sunburst (Autodesk Fusion 360 design; units mm, degrees)
Autodesk Fusion 360 part; units mm, degrees
extrude "Extrude6" [suppressed]
ref_plane "WorkPlane1" through (-0.7494, -0.6, 4.8151) normal (0, -1, 0) x (0, 0, -1)
sketch "Sketch3" plane through (0, -0.6, 0) normal (0, -1, 0) x (-1, 0, 0)
  circle A0 centre (0, 0) radius 28
  dimension "d32" = 56
  constraint coincident A0.centre origin
  measures "d32" diameter of A0
extrude "Extrude7" [suppressed]
sketch "sketch 197" plane through (0, 0, 0) normal (0, 1, 0) x (1, 0, 0)
  circle A0 centre (0, 0) radius 5
  circle A1 centre (0, 0) radius 6
  circle A2 centre (0, 0) radius 16
  circle A3 centre (0, 0) radius 17
  circle A4 centre (0, 0) radius 26.5
  circle A5 centre (0, 0) radius 27.5
  circle A6 centre (0, 0) radius 33
  line L0 (-3.9046, 4.5557) -> (-9.6929, 12.7298)
  line L1 (-5.6565, 2.001) -> (-15.1209, 5.2305)
  line L2 (-16.1216, 5.3938) -> (-25.1127, 8.4617)
  line L3 (-24.375, 10.3976) -> (-15.6425, 6.6566)
  line L4 (-15.4468, 7.0991) -> (-24.0905, 11.0407)
  line L5 (-15.0805, 7.8473) -> (-23.43, 12.3808)
  line L6 (-14.8296, 8.3116) -> (-23.1046, 12.9779)
  line L7 (-22.3505, 14.2374) -> (-14.3911, 9.0497)
  line L8 (-14.0817, 9.524) -> (-21.9358, 14.8684)
  line L9 (-20.5642, 16.7142) -> (-13.2548, 10.6447)
  line L10 (-26.5492, 7.1686) -> (-31.8756, 8.5408)
  line L11 (-31.236, 10.6447) -> (-26.0698, 8.7529)
  line L12 (-25.8745, 9.3144) -> (-31.0392, 11.2056)
  line L13 (-30.2541, 13.1791) -> (-25.2442, 10.9077)
  line L14 (-5.8159, 1.4749) -> (-15.3347, 4.5657)
  line L15 (-5.9819, -0.4663) -> (-15.8908, -1.8658)
  line L16 (-5.8856, -1.166) -> (-15.7623, -2.7475)
  line L17 (-3.2548, -5.0405) -> (-8.4775, -13.5695)
  line L18 (-7.87, -13.9307) -> (-2.6391, -5.3884)
  line L19 (0.3065, -5.9922) -> (1.4776, -15.9316)
  line L20 (2.4796, -15.8067) -> (1.09, -5.9002)
  line L21 (2.2431, -5.5649) -> (6.8423, -14.4632)
  line L22 (7.5569, -14.103) -> (2.964, -5.2168)
  line L23 (5.7898, 1.5741) -> (15.2163, 4.9462)
  line L24 (14.9323, 5.7469) -> (5.5751, 2.2176)
  line L25 (12.3522, 10.1697) -> (4.8981, 3.4653)
  line L26 (4.2215, 4.2636) -> (11.6613, 10.9551)
  line L27 (1.1172, 5.8951) -> (3.7964, 15.5431)
  line L28 (4.6866, 15.2982) -> (2.0085, 5.6538)
  line L29 (-3.1659, 5.0968) -> (-8.9039, 13.2936)
  line L30 (-16.5713, 3.7935) -> (-25.8898, 5.6538)
  line L31 (-16.3375, 4.6995) -> (-25.3936, 7.5771)
  line L32 (-26.399, 2.3114) -> (-16.9218, 1.6288)
  line L33 (-26.045, 4.8897) -> (-16.7279, 3.0296)
  line L34 (-26.4638, 1.3844) -> (-16.9855, 0.7017)
  line L35 (-26.2905, -3.3257) -> (-16.8977, -1.8621)
  line L36 (-26.191, -4.0353) -> (-16.7685, -2.7959)
  line L37 (-25.7871, -6.1054) -> (-16.5831, -3.742)
  line L38 (-7.4849, -25.421) -> (-4.6905, -16.3401)
  line L39 (-5.7669, -25.8649) -> (-3.8484, -16.5587)
  line L40 (0, -26.5) -> (0, -17)
  line L41 (-2.951, -16.7419) -> (-4.8696, -26.0487)
  line L42 (0.8661, -26.4858) -> (0.6304, -16.9883)
  line L43 (1.8311, -16.9011) -> (2.9765, -26.3323)
  line L44 (6.0603, -25.7977) -> (4.0068, -16.5211)
  line L45 (5.3634, -16.1318) -> (8.5144, -25.0949)
  line L46 (9.4324, -24.7645) -> (6.1019, -15.8672)
  line L47 (11.7605, -23.7474) -> (7.3572, -15.3255)
  line L48 (12.6046, -23.3104) -> (8.2022, -14.8904)
  line L49 (9.0465, -14.3931) -> (14.3256, -22.2941)
  line L50 (9.7988, -13.8918) -> (15.1912, -21.7135)
  line L51 (10.2957, -13.5277) -> (16.3371, -20.865)
  line L52 (11.0727, -12.8994) -> (17.1122, -20.2342)
  line L53 (11.8744, -12.1655) -> (18.6003, -18.8753)
  line L54 (13.7033, -10.0608) -> (21.1773, -15.9303)
  line L55 (15.9319, -5.9308) -> (24.934, -8.9747)
  line L56 (16.2213, -5.0862) -> (25.2771, -7.9572)
  line L57 (16.8901, -1.9298) -> (26.3655, -2.6665)
  line L58 (16.9669, -1.0605) -> (26.439, -1.797)
  line L59 (16.9902, 0.5773) -> (26.4772, 1.0989)
  line L60 (26.4135, 2.1398) -> (16.9358, 1.4761)
  line L61 (16.6138, 3.6031) -> (25.8333, 5.9067)
  line L62 (25.6212, 6.7677) -> (16.4033, 4.4645)
  line L63 (16.1363, 5.3498) -> (25.0535, 8.6356)
  line L64 (24.6784, 9.6554) -> (15.8245, 6.2117)
  line L65 (15.4197, 7.1577) -> (24.0445, 11.1406)
  line L66 (23.7354, 11.7848) -> (15.2099, 7.5934)
  line L67 (14.795, 8.373) -> (23.0554, 13.0652)
  line L68 (22.5, 14) -> (14.328, 9.1492)
  line L69 (21.2388, 15.8482) -> (13.553, 10.2623)
  line L70 (12.1982, 11.8408) -> (19.1494, 18.3181)
  line L71 (18.0736, 19.3803) -> (11.621, 12.4078)
  line L72 (11.1445, 12.8374) -> (17.6399, 19.7758)
  line L73 (16.0889, 21.057) -> (10.3305, 13.5011)
  line L74 (9.878, 13.8356) -> (15.6381, 21.3939)
  line L75 (14.6155, 22.1051) -> (9.3319, 14.2097)
  line L76 (7.3498, 15.3291) -> (11.7201, 23.7674)
  line L77 (9.9713, 24.5525) -> (6.3491, 15.7699)
  line L78 (9.2924, 24.8174) -> (5.8178, 15.9735)
  line L79 (7.4164, 25.4411) -> (4.7967, 16.3092)
  line L80 (6.3491, 25.7282) -> (3.8859, 16.5499)
  line L81 (3.8859, 26.2135) -> (2.6171, 16.7973)
  line L82 (3.1138, 26.3164) -> (1.8449, 16.8996)
  line L83 (1.2408, 26.4709) -> (0.92, 16.9751)
  line L84 (0.6334, 26.4924) -> (0.3127, 16.9971)
  line L85 (-1.1755, 26.4739) -> (-0.8096, 16.9807)
  line L86 (-1.8148, 26.4378) -> (-1.4486, 16.9382)
  line L87 (-4.2572, 26.1558) -> (-2.5895, 16.8016)
  line L88 (-4.9119, 26.0408) -> (-3.4233, 16.6518)
  line L89 (-6.7746, 25.6194) -> (-4.3029, 16.4464)
  line L90 (-7.4272, 25.4379) -> (-4.6925, 16.3395)
  line L91 (-8.6485, 25.049) -> (-5.5387, 16.0724)
  line L92 (-9.2604, 24.8293) -> (-5.9347, 15.9305)
  line L93 (-10.5439, 24.3121) -> (-6.7389, 15.6073)
  line L94 (-11.0798, 24.0726) -> (-7.2737, 15.3653)
  line L95 (-12.5073, 23.3627) -> (-8, 15)
  line L96 (-13.1462, 23.0093) -> (-8.446, 14.7535)
  line L97 (-15.2182, 21.6946) -> (-9.5864, 14.0392)
  line L98 (-15.9612, 21.1539) -> (-10.331, 13.5007)
  line L99 (-17.5978, 19.8133) -> (-11.2411, 12.7529)
  line L100 (-23.1855, 23.4826) -> (-19.2651, 19.6242)
  line L101 (-22.1696, 24.444) -> (-18.4895, 20.3566)
  line L102 (-21.5449, 24.9963) -> (-17.8638, 20.9078)
  line L103 (-20.5857, 25.792) -> (-17.0793, 21.5534)
  line L104 (-17.9748, 27.675) -> (-14.8657, 23.1357)
  line L105 (-16.2704, 28.7101) -> (-13.6536, 23.8711)
  line L106 (-15.7952, 28.9743) -> (-13.0339, 24.215)
  line L107 (-14.0759, 29.8474) -> (-11.7698, 24.854)
  line L108 (-10.616, 31.2458) -> (-8.8282, 26.0444)
  line L109 (-9.5266, 31.595) -> (-7.9766, 26.3178)
  line L110 (-8.6438, 31.8478) -> (-7.1988, 26.5411)
  line L111 (-7.5092, 32.1343) -> (-6.3363, 26.7601)
  line L112 (-0.704, 32.9925) -> (-0.5292, 27.4949)
  line L113 (0.5327, 32.9957) -> (0.4096, 27.4969)
  line L114 (1.4606, 32.9677) -> (1.1772, 27.4748)
  line L115 (2.6616, 32.8925) -> (2.1566, 27.4153)
  line L116 (13.4068, 30.1539) -> (11.1032, 25.1589)
  line L117 (12.255, 24.6184) -> (14.8392, 29.4754)
  line L118 (25.4963, 20.9509) -> (21.1963, 17.5204)
  line L119 (22.3915, 15.9647) -> (26.814, 19.2357)
  line L120 (30.5346, 12.5156) -> (25.4747, 10.3581)
  line L121 (25.8193, 9.4666) -> (30.9951, 11.3272)
  line L122 (31.7345, 9.0509) -> (26.4504, 7.5251)
  line L123 (26.7308, 6.4588) -> (32.0505, 7.8593)
  line L124 (32.5136, 5.6451) -> (27.1002, 4.6722)
  line L125 (27.2454, 3.7332) -> (32.6896, 4.5156)
  line L126 (32.7629, 3.9486) -> (27.2995, 3.3149)
  line L127 (27.3861, 2.5002) -> (32.8643, 2.9897)
  line L128 (32.9337, 2.0913) -> (27.4395, 1.8225)
  line L129 (27.4849, 0.9123) -> (32.9874, 0.9123)
  line L130 (32.9822, -1.085) -> (27.4849, -0.9117)
  line L131 (27.4395, -1.8225) -> (32.9306, -2.1396)
  line L132 (32.7757, -3.8411) -> (27.3199, -3.1425)
  line L133 (27.1875, -4.1342) -> (32.6082, -5.07)
  line L134 (5.5375, -32.5321) -> (4.6, -27.1125)
  line L135 (3.5952, -27.264) -> (4.2286, -32.728)
  line L136 (3.0895, -27.3259) -> (3.6634, -32.796)
  line L137 (2.669, -32.8919) -> (2.3996, -27.3951)
  line L138 (2.2276, -32.9247) -> (1.8643, -27.4367)
  line L139 (1.2645, -32.9758) -> (1.0932, -27.4783)
  line L140 (0.7707, -32.991) -> (0.5994, -27.4935)
  line L141 (-0.9829, -32.9854) -> (-0.8607, -27.4865)
  line L142 (-1.7716, -32.9524) -> (-1.5108, -27.4585)
  line L143 (-4.0581, -32.7495) -> (-3.3505, -27.2951)
  line L144 (-30.3823, -12.8808) -> (-25.4093, -10.5174)
  line L145 (-26.1354, -8.5552) -> (-31.4006, -10.1491)
  line L146 (-26.3937, -7.7215) -> (-31.6471, -9.3522)
  line L147 (-26.6921, -6.6169) -> (-32.0193, -7.9853)
  line L148 (-26.8427, -5.9766) -> (-32.2121, -7.1681)
  line L149 (-27.1016, -4.6639) -> (-32.5055, -5.6915)
  constraint coincident A0.centre A1.centre
  constraint concentric A0 A1
  constraint concentric A1 A2
  constraint concentric A1 A3
  constraint concentric A3 A5
  constraint concentric A4 A6
  constraint coincident A1 L0.start
  constraint coincident A2 L0.end
  constraint coincident A1 L1.start
  constraint coincident A2 L1.end
  constraint coincident A3 L2.start
  constraint coincident A4 L2.end
  constraint parallel L1 L2
  constraint coincident A4 L3.start
  constraint coincident A3 L3.end
  constraint coincident A3 L4.start
  constraint coincident A4 L4.end
  constraint coincident A3 L5.start
  constraint coincident A4 L5.end
  constraint coincident A3 L6.start
  constraint coincident A4 L6.end
  constraint coincident A4 L7.start
  constraint coincident A3 L7.end
  constraint coincident A3 L8.start
  constraint coincident A4 L8.end
  constraint coincident A4 L9.start
  constraint coincident A3 L9.end
  constraint coincident A5 L10.start
  constraint coincident A6 L10.end
  constraint coincident A6 L11.start
  constraint coincident A5 L11.end
  constraint coincident A5 L12.start
  constraint coincident A6 L12.end
  constraint parallel L11 L12
  constraint coincident A6 L13.start
  constraint coincident A5 L13.end
  constraint coincident A1 L14.start
  constraint coincident A2 L14.end
  constraint coincident A1 L15.start
  constraint coincident A2 L15.end
  constraint coincident A1 L16.start
  constraint coincident A2 L16.end
  constraint coincident A1 L17.start
  constraint coincident A2 L17.end
  constraint coincident A2 L18.start
  constraint coincident A1 L18.end
  constraint parallel L17 L18
  constraint coincident A1 L19.start
  constraint coincident A2 L19.end
  constraint coincident A2 L20.start
  constraint coincident A1 L20.end
  constraint coincident A1 L21.start
  constraint coincident A2 L21.end
  constraint coincident A2 L22.start
  constraint coincident A1 L22.end
  constraint parallel L21 L22
  constraint coincident A1 L23.start
  constraint coincident A2 L23.end
  constraint coincident A2 L24.start
  constraint coincident A1 L24.end
  constraint coincident A2 L25.start
  constraint coincident A1 L25.end
  constraint coincident A1 L26.start
  constraint coincident A2 L26.end
  constraint parallel L25 L26
  constraint coincident A1 L27.start
  constraint coincident A2 L27.end
  constraint coincident A2 L28.start
  constraint coincident A1 L28.end
  constraint parallel L27 L28
  constraint coincident A1 L29.start
  constraint coincident A2 L29.end
  constraint coincident A3 L30.start
  constraint coincident A4 L30.end
  constraint coincident A3 L31.start
  constraint coincident A4 L31.end
  constraint coincident A4 L32.start
  constraint coincident A3 L32.end
  constraint coincident A4 L33.start
  constraint coincident A3 L33.end
  constraint parallel L30 L33
  constraint coincident A4 L34.start
  constraint coincident A3 L34.end
  constraint parallel L32 L34
  constraint coincident A4 L35.start
  constraint coincident A3 L35.end
  constraint coincident A4 L36.start
  constraint coincident A3 L36.end
  constraint coincident A4 L37.start
  constraint coincident A3 L37.end
  constraint coincident A4 L38.start
  constraint coincident A3 L38.end
  constraint coincident A4 L39.start
  constraint coincident A3 L39.end
  constraint coincident A4 L40.start
  constraint coincident A3 L40.end
  constraint vertical L40
  constraint coincident A3 L41.start
  constraint coincident A4 L41.end
  constraint parallel L39 L41
  constraint coincident A4 L42.start
  constraint coincident A3 L42.end
  constraint coincident A3 L43.start
  constraint coincident A4 L43.end
  constraint coincident A4 L44.start
  constraint coincident A3 L44.end
  constraint coincident A3 L45.start
  constraint coincident A4 L45.end
  constraint coincident A4 L46.start
  constraint coincident A3 L46.end
  constraint coincident A4 L47.start
  constraint coincident A3 L47.end
  constraint coincident A4 L48.start
  constraint coincident A3 L48.end
  constraint parallel L47 L48
  constraint coincident A3 L49.start
  constraint coincident A4 L49.end
  constraint coincident A3 L50.start
  constraint coincident A4 L50.end
  constraint coincident A3 L51.start
  constraint coincident A4 L51.end
  constraint coincident A3 L52.start
  constraint coincident A4 L52.end
  constraint parallel L51 L52
  constraint coincident A3 L53.start
  constraint coincident A4 L53.end
  constraint coincident A3 L54.start
  constraint coincident A4 L54.end
  constraint coincident A3 L55.start
  constraint coincident A4 L55.end
  constraint coincident A3 L56.start
  constraint coincident A4 L56.end
  constraint coincident A3 L57.start
  constraint coincident A4 L57.end
  constraint coincident A3 L58.start
  constraint coincident A4 L58.end
  constraint parallel L57 L58
  constraint coincident A3 L59.start
  constraint coincident A4 L59.end
  constraint coincident A3 L60.end
  constraint coincident A3 L61.start
  constraint coincident A4 L61.end
  constraint coincident A4 L62.start
  constraint coincident A3 L62.end
  constraint parallel L61 L62
  constraint coincident A3 L63.start
  constraint coincident A4 L63.end
  constraint coincident A4 L64.start
  constraint coincident A3 L64.end
  constraint coincident A3 L65.start
  constraint coincident A4 L65.end
  constraint coincident A4 L66.start
  constraint coincident A3 L66.end
  constraint coincident A3 L67.start
  constraint coincident A4 L67.end
  constraint coincident A4 L68.start
  constraint coincident A3 L68.end
  constraint coincident A4 L69.start
  constraint coincident A3 L69.end
  constraint coincident A3 L70.start
  constraint coincident A4 L70.end
  constraint coincident A4 L71.start
  constraint coincident A3 L71.end
  constraint coincident A3 L72.start
  constraint coincident A4 L72.end
  constraint coincident A4 L73.start
  constraint coincident A3 L73.end
  constraint coincident A3 L74.start
  constraint coincident A4 L74.end
  constraint parallel L73 L74
  constraint coincident A4 L75.start
  constraint coincident A3 L75.end
  constraint coincident A3 L76.start
  constraint coincident A4 L76.end
  constraint coincident A4 L77.start
  constraint coincident A3 L77.end
  constraint coincident A4 L78.start
  constraint coincident A3 L78.end
  constraint coincident A4 L79.start
  constraint coincident A3 L79.end
  constraint coincident A4 L80.start
  constraint coincident A3 L80.end
  constraint coincident A4 L81.start
  constraint coincident A3 L81.end
  constraint coincident A4 L82.start
  constraint coincident A3 L82.end
  constraint parallel L81 L82
  constraint coincident A4 L83.start
  constraint coincident A3 L83.end
  constraint coincident A4 L84.start
  constraint coincident A3 L84.end
  constraint parallel L83 L84
  constraint coincident A4 L85.start
  constraint coincident A3 L85.end
  constraint coincident A4 L86.start
  constraint coincident A3 L86.end
  constraint parallel L85 L86
  constraint coincident A4 L87.start
  constraint coincident A3 L87.end
  constraint coincident A4 L88.start
  constraint coincident A3 L88.end
  constraint coincident A4 L89.start
  constraint coincident A3 L89.end
  constraint coincident A4 L90.start
  constraint coincident A3 L90.end
  constraint coincident A4 L91.start
  constraint coincident A3 L91.end
  constraint coincident A4 L92.start
  constraint coincident A3 L92.end
  constraint coincident A4 L93.start
  constraint coincident A3 L93.end
  constraint coincident A4 L94.start
  constraint coincident A3 L94.end
  constraint parallel L93 L94
  constraint coincident A4 L95.start
  constraint coincident A3 L95.end
  constraint coincident A4 L96.start
  constraint coincident A3 L96.end
  constraint coincident A4 L97.start
  constraint coincident A3 L97.end
  constraint coincident A4 L98.start
  constraint coincident A3 L98.end
  constraint parallel L97 L98
  constraint coincident A4 L99.start
  constraint coincident A3 L99.end
  constraint coincident A6 L100.start
  constraint coincident A5 L100.end
  constraint coincident A6 L101.start
  constraint coincident A5 L101.end
  constraint parallel L99 L101
  constraint coincident A6 L102.start
  constraint coincident A5 L102.end
  constraint parallel L101 L102
  constraint coincident A6 L103.start
  constraint coincident A5 L103.end
  constraint coincident A6 L104.start
  constraint coincident A5 L104.end
  constraint coincident A6 L105.start
  constraint coincident A5 L105.end
  constraint coincident A6 L106.start
  constraint coincident A5 L106.end
  constraint coincident A6 L107.start
  constraint coincident A5 L107.end
  constraint coincident A6 L108.start
  constraint coincident A5 L108.end
  constraint coincident A6 L109.start
  constraint coincident A5 L109.end
  constraint coincident A6 L110.start
  constraint coincident A5 L110.end
  constraint coincident A6 L111.start
  constraint coincident A5 L111.end
  constraint coincident A6 L112.start
  constraint coincident A5 L112.end
  constraint coincident A6 L113.start
  constraint coincident A5 L113.end
  constraint coincident A6 L114.start
  constraint coincident A5 L114.end
  constraint coincident A6 L115.start
  constraint coincident A5 L115.end
  constraint coincident A6 L116.start
  constraint coincident A5 L116.end
  constraint coincident A5 L117.start
  constraint coincident A6 L117.end
  constraint coincident A6 L118.start
  constraint coincident A5 L118.end
  constraint coincident A5 L119.start
  constraint coincident A6 L119.end
  constraint coincident A6 L120.start
  constraint coincident A5 L120.end
  constraint coincident A5 L121.start
  constraint coincident A6 L121.end
  constraint coincident A6 L122.start
  constraint coincident A5 L122.end
  constraint coincident A5 L123.start
  constraint coincident A6 L123.end
  constraint coincident A6 L124.start
  constraint coincident A5 L124.end
  constraint coincident A5 L125.start
  constraint coincident A6 L125.end
  constraint coincident A6 L126.start
  constraint coincident A5 L126.end
  constraint coincident A5 L127.start
  constraint coincident A6 L127.end
  constraint coincident A6 L128.start
  constraint coincident A5 L128.end
  constraint coincident A6 L129.end
  constraint horizontal L129
  constraint coincident A6 L130.start
  constraint coincident A5 L130.end
  constraint coincident A5 L131.start
  constraint coincident A6 L131.end
  constraint coincident A6 L132.start
  constraint coincident A5 L132.end
  constraint coincident A5 L133.start
  constraint coincident A6 L133.end
  constraint coincident A6 L134.start
  constraint coincident A5 L134.end
  constraint coincident A5 L135.start
  constraint coincident A6 L135.end
  constraint coincident A5 L136.start
  constraint coincident A6 L136.end
  constraint coincident A6 L137.start
  constraint coincident A5 L137.end
  constraint coincident A6 L138.start
  constraint coincident A5 L138.end
  constraint coincident A6 L139.start
  constraint coincident A5 L139.end
  constraint coincident A6 L140.start
  constraint coincident A5 L140.end
  constraint parallel L139 L140
  constraint coincident A5 L141.end
  constraint coincident A6 L142.start
  constraint coincident A5 L142.end
  constraint coincident A6 L143.start
  constraint coincident A5 L143.end
  constraint coincident A6 L144.start
  constraint coincident A5 L144.end
  constraint coincident A5 L145.start
  constraint coincident A6 L145.end
  constraint coincident A5 L146.start
  constraint coincident A6 L146.end
  constraint coincident A5 L147.start
  constraint coincident A6 L147.end
  constraint coincident A5 L148.start
  constraint coincident A6 L148.end
  constraint coincident A5 L149.start
  constraint coincident A6 L149.end
  constraint coincident A6 L141.start
  constraint coincident A5 L129.start
  constraint coincident A4 L60.start
  measures "d1" diameter of A0
  measures "d2" diameter of A1
  measures "d3" diameter of A2
  measures "d4" diameter of A3
  measures "d5" diameter of A4
  measures "d6" diameter of A5
  measures "d7" diameter of A6
extrude "Extrude8" add sketch "sketch 197" against normal blind 1.8 contours A0 | A1 | A1 A2 L22 L23 | A1 A2 L23 L24 | A1 A2 L21 L22 | A1 A2 L24 L25 | A1 A2 L20 L21 | A1 A2 L25 L26 | A1 A2 L19 L20 | A1 A2 L26 L28 | A1 A2 L18 L19 | A1 A2 L27 L28 | A1 A2 L17 L18 | A1 A2 L27 L29 | A1 A2 L16 L17 | A1 A2 L0 L29 | A1 A2 L15 L16 | A1 A2 L0 L1 | A1 A2 L14 L15 | A1 A2 L1 L14 | A3 | A3 A4 L58 L59 | A3 A4 L59 L60 | A3 A4 L57 L58 | A3 A4 L60 L61 | A3 A4 L56 L57 | A3 A4 L61 L62 | A3 A4 L55 L56 | A3 A4 L62 L63 | A3 A4 L54 L55 | A3 A4 L63 L64 | A3 A4 L53 L54 | A3 A4 L64 L65 | A3 A4 L52 L53 | A3 A4 L65 L66 | A3 A4 L51 L52 | A3 A4 L66 L67 | A3 A4 L50 L51 | A3 A4 L67 L68 | A3 A4 L49 L50 | A3 A4 L68 L69 | A3 A4 L48 L49 | A3 A4 L69 L70 | A3 A4 L47 L48 | A3 A4 L70 L71 | A3 A4 L46 L47 | A3 A4 L71 L72 | A3 A4 L45 L46 | A3 A4 L72 L73 | A3 A4 L44 L45 | A3 A4 L73 L74 | A3 A4 L43 L44 | A3 A4 L74 L75 | A3 A4 L42 L43 | A3 A4 L75 L76 | A3 A4 L40 L42 | A3 A4 L76 L77 | A3 A4 L40 L41 | A3 A4 L77 L78 | A3 A4 L39 L41 | A3 A4 L78 L79 | A3 A4 L38 L39 | A3 A4 L79 L80 | A3 A4 L37 L38 | A3 A4 L80 L81 | A3 A4 L36 L37 | A3 A4 L81 L82 | A3 A4 L35 L36 | A3 A4 L82 L83 | A3 A4 L34 L35 | A3 A4 L83 L84 | A3 A4 L32 L34 | A3 A4 L84 L85 | A3 A4 L32 L33 | A3 A4 L85 L86 | A3 A4 L30 L33 | A3 A4 L86 L87 | A3 A4 L30 L31 | A3 A4 L87 L88 | A3 A4 L2 L31 | A3 A4 L88 L89 | A3 A4 L2 L3 | A3 A4 L89 L90 | A3 A4 L3 L4 | A3 A4 L90 L91 | A3 A4 L4 L5 | A3 A4 L91 L92 | A3 A4 L5 L6 | A3 A4 L92 L93 | A3 A4 L6 L7 | A3 A4 L93 L94 | A3 A4 L7 L8 | A3 A4 L94 L95 | A3 A4 L8 L9 | A3 A4 L95 L96 | A3 A4 L9 L99 | A3 A4 L96 L97 | A3 A4 L98 L99 | A3 A4 L97 L98 | A5 | A5 A6 L129 L130 | A5 A6 L128 L129 | A5 A6 L130 L131 | A5 A6 L127 L128 | A5 A6 L131 L132 | A5 A6 L126 L127 | A5 A6 L132 L133 | A5 A6 L125 L126 | A5 A6 L133 L134 | A5 A6 L124 L125 | A5 A6 L134 L135 | A5 A6 L123 L124 | A5 A6 L135 L136 | A5 A6 L122 L123 | A5 A6 L136 L137 | A5 A6 L121 L122 | A5 A6 L137 L138 | A5 A6 L120 L121 | A5 A6 L138 L139 | A5 A6 L119 L120 | A5 A6 L139 L140 | A5 A6 L118 L119 | A5 A6 L140 L141 | A5 A6 L117 L118 | A5 A6 L141 L142 | A5 A6 L116 L117 | A5 A6 L142 L143 | A5 A6 L115 L116 | A5 A6 L143 L144 | A5 A6 L114 L115 | A5 A6 L144 L145 | A5 A6 L113 L114 | A5 A6 L145 L146 | A5 A6 L112 L113 | A5 A6 L146 L147 | A5 A6 L111 L112 | A5 A6 L147 L148 | A5 A6 L110 L111 | A5 A6 L148 L149 | A5 A6 L109 L110 | A5 A6 L10 L149 | A5 A6 L108 L109 | A5 A6 L10 L11 | A5 A6 L107 L108 | A5 A6 L11 L12 | A5 A6 L106 L107 | A5 A6 L12 L13 | A5 A6 L105 L106 | A5 A6 L13 L100 | A5 A6 L104 L105 | A5 A6 L100 L101 | A5 A6 L103 L104 | A5 A6 L101 L102 | A5 A6 L102 L103 makes body 1
extrude "Extrude1" add sketch "sketch 197" along normal blind 1 separate body contours A1 A2 L18 L19 | A1 A2 L27 L29 | A1 A2 L16 L17 | A1 A2 L0 L1 | A1 A2 L14 L15 makes body 2 at (-12.3205, 0, -2.8314) makes body 3 at (-12.2909, 0, 2.9444) makes body 4 at (-8.3492, 0, -9.4871) makes body 5 at (-5.545, 0, 11.3667) makes body 6 at (-1.347, 0, -12.5692) in component "Ring 0 - pro"
extrude "Extrude1'" add sketch "sketch 197" along normal blind 1 separate body contours A1 A2 L22 L23 | A1 A2 L24 L25 | A1 A2 L20 L21 | A1 A2 L26 L28 makes body 7 at (12.451, 0, 2.1821) makes body 8 at (10.9191, 0, -6.3897) makes body 9 at (4.8395, 0, 11.6925) makes body 10 at (5.9656, 0, -11.1484) in component "Ring 0 - con"
extrude "Extrude1''" add sketch "sketch 197" along normal blind 0.8 separate body contours A3 A4 L58 L59 | A3 A4 L60 L61 | A3 A4 L66 L67 | A3 A4 L68 L69 | A3 A4 L46 L47 | A3 A4 L42 L43 | A3 A4 L76 L77 | A3 A4 L40 L41 | A3 A4 L78 L79 | A3 A4 L36 L37 | A3 A4 L34 L35 | A3 A4 L32 L33 | A3 A4 L88 L89 | A3 A4 L2 L3 | A3 A4 L90 L91 | A3 A4 L4 L5 | A3 A4 L92 L93 | A3 A4 L6 L7 | A3 A4 L94 L95 | A3 A4 L8 L9 | A3 A4 L96 L97 makes body 11 at (-23.21, 0, -2.3716) makes body 12 at (-18.286, 0, -14.4904) makes body 13 at (-6.7465, 0, -22.3361) makes body 14 at (19.6417, 0, -12.5923) makes body 15 at (10.0377, 0, 21.0614) makes body 16 at (2.3607, 0, 23.2119) makes body 17 at (20.8206, 0, -10.5313) makes body 18 at (-5.137, 0, -22.7595) makes body 19 at (-13.1153, 0, -19.296) makes body 20 at (-21.9898, 0, -7.798) makes body 21 at (-23.2099, 0, 2.3159) makes body 22 at (-19.7838, 0, -12.3698) makes body 23 at (-9.134, 0, -21.4704) makes body 24 at (10.0711, 0, -21.0465) makes body 25 at (23.3224, 0, -0.6032) makes body 26 at (-3.6924, 0, 23.0299) makes body 27 at (22.8447, 0, -4.7235) makes body 28 at (7.9275, 0, -21.9439) makes body 29 at (-9.9713, 0, -21.0945) makes body 30 at (-20.723, 0, -10.7221) makes body 31 at (-23.0114, 0, 3.8533) in component "Ring 1 - pro"
extrude "Extrude1'''" add sketch "sketch 197" along normal blind 0.8 separate body contours A3 A4 L56 L57 | A3 A4 L62 L63 | A3 A4 L54 L55 | A3 A4 L64 L65 | A3 A4 L52 L53 | A3 A4 L50 L51 | A3 A4 L48 L49 | A3 A4 L70 L71 | A3 A4 L72 L73 | A3 A4 L44 L45 | A3 A4 L74 L75 | A3 A4 L38 L39 | A3 A4 L80 L81 | A3 A4 L82 L83 | A3 A4 L84 L85 | A3 A4 L86 L87 | A3 A4 L30 L31 | A3 A4 L98 L99 makes body 32 at (-1.965, 0, -23.2483) makes body 33 at (13.3196, 0, -19.1575) makes body 34 at (22.1492, 0, -7.3344) makes body 35 at (13.89, 0, 18.7478) makes body 36 at (-5.3194, 0, 22.7178) makes body 37 at (15.2682, 0, 17.6425) makes body 38 at (21.66, 0, -8.6739) makes body 39 at (5.2561, 0, -22.7313) makes body 40 at (-14.2703, 0, -18.4588) makes body 41 at (0.3255, 0, -23.3298) makes body 42 at (15.3061, 0, -17.6097) makes body 43 at (23.1262, 0, 3.0166) makes body 44 at (12.3775, 0, 19.7782) makes body 45 at (5.651, 0, 22.6362) makes body 46 at (19.1799, 0, 13.244) makes body 47 at (16.715, 0, -16.2793) makes body 48 at (2.4832, 0, -23.1996) makes body 49 at (-22.7339, 0, -5.2488) in component "Ring 1 - con"
extrude "Extrude1''''" add sketch "sketch 197" along normal blind 0.4 separate body contours A5 A6 L128 L129 | A5 A6 L130 L131 | A5 A6 L134 L135 | A5 A6 L136 L137 | A5 A6 L118 L119 | A5 A6 L114 L115 | A5 A6 L112 L113 | A5 A6 L146 L147 | A5 A6 L148 L149 | A5 A6 L10 L11 | A5 A6 L12 L13 makes body 50 at (25.0689, 0, -18.5151) makes body 51 at (-29.5902, 0, -9.782) makes body 52 at (4.1632, 0, 30.8868) makes body 53 at (-30.6477, 0, 5.6598) makes body 54 at (2.36, 0, -31.0767) makes body 55 at (31.1488, 0, -1.0434) makes body 56 at (-28.6761, 0, -12.2046) makes body 57 at (2.9876, 0, 31.0229) makes body 58 at (-29.9395, 0, 8.6573) makes body 59 at (-0.5083, 0, -31.162) makes body 60 at (31.1134, 0, 1.8156) in component "Ring 2 - pro"
extrude "Extrude1'''''" add sketch "sketch 197" along normal blind 0.4 separate body contours A5 A6 L126 L127 | A5 A6 L132 L133 | A5 A6 L124 L125 | A5 A6 L122 L123 | A5 A6 L120 L121 | A5 A6 L138 L139 | A5 A6 L140 L141 | A5 A6 L116 L117 | A5 A6 L142 L143 | A5 A6 L144 L145 | A5 A6 L110 L111 | A5 A6 L108 L109 | A5 A6 L106 L107 | A5 A6 L104 L105 | A5 A6 L100 L101 | A5 A6 L102 L103 makes body 61 at (30.7301, 0, -5.1955) makes body 62 at (-7.2447, 0, -30.3125) makes body 63 at (-20.2124, 0, -23.7232) makes body 64 at (0.5188, 0, 31.1613) makes body 65 at (-1.9392, 0, 31.1045) makes body 66 at (-16.7514, 0, -26.2807) makes body 67 at (13.8199, 0, -27.9343) makes body 68 at (30.9646, 0, -3.5405) makes body 69 at (30.2142, 0, -7.6442) makes body 70 at (-9.1314, 0, -29.7985) makes body 71 at (-21.7673, 0, -22.3049) makes body 72 at (1.3145, 0, 31.1386) makes body 73 at (-28.8467, 0, 11.7929) makes body 74 at (-14.6856, 0, -27.4886) makes body 75 at (28.9008, 0, -11.665) makes body 76 at (30.8216, 0, 4.6217) in component "Ring 2 - con"
extrude "Extrude1''''''" add sketch "sketch 197" along normal blind 1.2 separate body contours A0 makes body 77 in component "Thesis"
sketch "sketch 6374" plane through (0, -1.2, 0) normal (0, -1, 0) x (1, 0, 0)
  circle A0 centre (0, 0) radius 33
  line L0 (0, 0) -> (-33, 0)
  circle A1 centre (0, 0) radius 4.5
  circle A2 centre (0, 0) radius 6
  circle A3 centre (0, 0) radius 7.5
  circle A4 centre (0, 0) radius 9
  circle A5 centre (0, 0) radius 12
  circle A6 centre (0, 0) radius 10.5
  line L1 (0, 0) -> (9.8298, -6.8829)
  line L2 (0, 0) -> (-9.8298, -6.8829)
  line L3 (3.6862, -2.5811) -> (0, 0)
  line L4 (4.9149, -3.4415) -> (0, 0)
  line L5 (6.1436, -4.3018) -> (0, 0)
  line L6 (7.3724, -5.1622) -> (0, 0)
  line L7 (8.6011, -6.0226) -> (0, 0)
  line L8 (-3.6862, -2.5811) -> (0, 0)
  line L9 (-4.9149, -3.4415) -> (0, 0)
  line L10 (0, 0) -> (-6.1436, -4.3018)
  line L11 (0, 0) -> (-7.3724, -5.1622)
  line L12 (0, 0) -> (-8.6011, -6.0226)
  arc A7 (9.8298, -6.8829) -> (8.6011, -6.0226) centre (9.2155, -6.4527) ccw
  arc A8 (7.3724, -5.1622) -> (6.1436, -4.3018) centre (6.758, -4.732) ccw
  arc A9 (4.9149, -3.4415) -> (3.6862, -2.5811) centre (4.3005, -3.0113) ccw
  arc A10 (-3.6862, -2.5811) -> (-4.9149, -3.4415) centre (-4.3005, -3.0113) ccw
  arc A11 (-6.1436, -4.3018) -> (-7.3724, -5.1622) centre (-6.758, -4.732) ccw
  arc A12 (-8.6011, -6.0226) -> (-9.8298, -6.8829) centre (-9.2155, -6.4527) ccw
  line L13 (11.8052, 0.0152) -> (10.0886, 0.0152)
  line L14 (10.0886, 0.0152) -> (5.9554, 7.4033)
  line L15 (5.9554, 7.4033) -> (6.1139, 7.575)
  line L16 (6.1139, 7.575) -> (6.1139, 0.0152)
  line L17 (6.1139, 0.0152) -> (4.5821, 0.0152)
  line L18 (4.5821, 0.0152) -> (4.5821, 9.6085)
  line L19 (4.5821, 9.6085) -> (6.312, 9.6085)
  line L20 (6.312, 9.6085) -> (10.4319, 2.3326)
  line L21 (10.4319, 2.3326) -> (10.2735, 2.161)
  line L22 (10.2735, 2.161) -> (10.2735, 9.6085)
  line L23 (10.2735, 9.6085) -> (11.8052, 9.6085)
  line L24 (11.8052, 9.6085) -> (11.8052, 0.0152)
  line L25 (2.3373, 0.0152) -> (0.7593, 0.0152)
  line L26 (0.7593, 0.0152) -> (0.7593, 9.6151)
  line L27 (0.7593, 9.6151) -> (2.3373, 9.6151)
  line L28 (2.3373, 9.6151) -> (2.3373, 0.0152)
  line L29 (1.677, 4.1747) -> (-3.1098, 4.1747)
  line L30 (-3.1098, 4.1747) -> (-3.1098, 5.6867)
  line L31 (-3.1098, 5.6867) -> (1.677, 5.6867)
  line L32 (1.677, 5.6867) -> (1.677, 4.1747)
  line L33 (1.677, 0.0152) -> (-3.836, 0.0152)
  line L34 (-3.836, 0.0152) -> (-3.836, 1.5271)
  line L35 (-3.836, 1.5271) -> (1.677, 1.5271)
  line L36 (1.677, 1.5271) -> (1.677, 0.0152)
  spline S0 degree 2 poles (-8.4314, 9.7142) (-7.3882, 9.7142) (-6.619, 9.2817) knots 0 0 0 1 1 1
  spline S1 degree 2 poles (-6.619, 9.2817) (-5.8498, 8.8493) (-5.4371, 8.0438) knots 0 0 0 1 1 1
  spline S2 degree 2 poles (-5.4371, 8.0438) (-5.0245, 7.2383) (-5.0245, 6.1356) knots 0 0 0 1 1 1
  line L37 (-5.0245, 6.1356) -> (-5.0245, 3.5013)
  spline S3 degree 2 poles (-5.0245, 3.5013) (-5.0245, 2.3986) (-5.4371, 1.5898) knots 0 0 0 1 1 1
  spline S4 degree 2 poles (-5.4371, 1.5898) (-5.8498, 0.781) (-6.619, 0.3486) knots 0 0 0 1 1 1
  spline S5 degree 2 poles (-6.619, 0.3486) (-7.3882, -0.0839) (-8.4314, -0.0839) knots 0 0 0 1 1 1
  spline S6 degree 2 poles (-8.4314, -0.0839) (-9.2963, -0.0839) (-9.9994, 0.2859) knots 0 0 0 1 1 1
  spline S7 degree 2 poles (-9.9994, 0.2859) (-10.7026, 0.6556) (-11.1681, 1.3522) knots 0 0 0 1 1 1
  spline S8 degree 2 poles (-11.1681, 1.3522) (-11.6336, 2.0487) (-11.8052, 2.9995) knots 0 0 0 1 1 1
  line L38 (-11.8052, 2.9995) -> (-10.181, 2.9995)
  spline S9 degree 2 poles (-10.181, 2.9995) (-10.0622, 2.5373) (-9.8047, 2.1907) knots 0 0 0 1 1 1
  spline S10 degree 2 poles (-9.8047, 2.1907) (-9.5472, 1.844) (-9.1939, 1.6592) knots 0 0 0 1 1 1
  spline S11 degree 2 poles (-9.1939, 1.6592) (-8.8407, 1.4743) (-8.4314, 1.4743) knots 0 0 0 1 1 1
  spline S12 degree 2 poles (-8.4314, 1.4743) (-7.8834, 1.4743) (-7.4839, 1.7219) knots 0 0 0 1 1 1
  spline S13 degree 2 poles (-7.4839, 1.7219) (-7.0845, 1.9695) (-6.8699, 2.4251) knots 0 0 0 1 1 1
  spline S14 degree 2 poles (-6.8699, 2.4251) (-6.6553, 2.8806) (-6.6553, 3.5013) knots 0 0 0 1 1 1
  line L39 (-6.6553, 3.5013) -> (-6.6553, 6.1356)
  spline S15 degree 2 poles (-6.6553, 6.1356) (-6.6553, 6.7497) (-6.8699, 7.2052) knots 0 0 0 1 1 1
  spline S16 degree 2 poles (-6.8699, 7.2052) (-7.0845, 7.6608) (-7.4839, 7.9051) knots 0 0 0 1 1 1
  spline S17 degree 2 poles (-7.4839, 7.9051) (-7.8834, 8.1494) (-8.4314, 8.1494) knots 0 0 0 1 1 1
  spline S18 degree 2 poles (-8.4314, 8.1494) (-8.8473, 8.1494) (-9.2005, 7.9744) knots 0 0 0 1 1 1
  spline S19 degree 2 poles (-9.2005, 7.9744) (-9.5538, 7.7995) (-9.8113, 7.4561) knots 0 0 0 1 1 1
  spline S20 degree 2 poles (-9.8113, 7.4561) (-10.0688, 7.1128) (-10.181, 6.6308) knots 0 0 0 1 1 1
  line L40 (-10.181, 6.6308) -> (-11.8052, 6.6308)
  spline S21 degree 2 poles (-11.8052, 6.6308) (-11.6336, 7.5816) (-11.1648, 8.2748) knots 0 0 0 1 1 1
  spline S22 degree 2 poles (-11.1648, 8.2748) (-10.696, 8.9681) (-9.9961, 9.3411) knots 0 0 0 1 1 1
  spline S23 degree 2 poles (-9.9961, 9.3411) (-9.2963, 9.7142) (-8.4314, 9.7142) knots 0 0 0 1 1 1
  circle A13 centre (0, 0) radius 33
  constraint coincident A0.centre L0.start
  constraint coincident A0 L0.end
  constraint horizontal L0
  constraint concentric A0 A1
  constraint concentric A2 A4
  constraint concentric A3 A5
  constraint concentric A0 A6
  constraint coincident A5 L1.end
  constraint coincident A5 L2.end
  constraint coincident L1 L3.start
  constraint coincident A1 L3.start
  constraint midpoint L1 L4.start
  constraint coincident L1 L5.start
  constraint coincident A3 L5.start
  constraint coincident L1 L6.start
  constraint coincident A4 L6.start
  constraint coincident L1 L7.start
  constraint coincident A6 L7.start
  constraint coincident A1 L8.start
  constraint coincident L2 L8.start
  constraint midpoint L2 L9.start
  constraint coincident L2 L10.end
  constraint coincident A3 L10.end
  constraint coincident A4 L11.end
  constraint coincident L2 L11.end
  constraint coincident A6 L12.end
  constraint coincident L2 L12.end
  constraint coincident L1 A7.centre
  constraint coincident L1 A8.centre
  constraint coincident L6 A9.centre
  constraint coincident L11 A11.centre
  constraint coincident L10 A10.centre
  constraint coincident L2 A12.centre
  measures "d21" diameter of A5
  measures "d22" diameter of A6
  measures "d23" diameter of A4
  measures "d24" diameter of A3
  measures "d25" diameter of A2
  measures "d26" diameter of A1
  measures "d28" angle of L0 L1
extrude "Extrude11" cut sketch "sketch 6374" against normal blind 0.15 from surface at 0.6 contours A1 A2 L1 L2 L4 L5 L6 L7 L9 L10 L11 L12 | L1 L4 L5 L6 L7 A9 | L2 L9 L10 L11 L12 A10 | A1 A2 L26 L29 L30 L31 | A1 L26 L29 | A2 A3 L37 S3 S4 S5 S13 S14 | A2 S3 S4 | A1 L26 L31 L32 | A1 L26 L29 L32 | A1 L25 L26 L28 L29 L32 L35 L36 | A1 A2 L26 L28 L31 L32 | A3 A4 L1 L2 L6 L7 L11 L12 | L1 L6 L7 A8 | L2 L11 L12 A11 | L0 A4 S5 S6 | L0 A3 A4 S5 S11 S12 S13 | L25 L26 L33 L35 L36 | L26 L33 L34 L35 | A2 L30 L31 | A2 A3 L26 L28 | A2 L17 L18 | A2 A3 L16 L17 L18 | L0 A4 S6 | L0 A4 A6 S6 S7 S9 S10 S11 | A3 A4 L26 L28 | A3 A4 L16 L18 | A5 A6 L1 L2 | L1 A7 | L2 A12 | A3 A4 S2 L37 S14 L39 | A4 L26 L27 L28 | L14 L15 L16 | A4 A6 L13 L14 L16 L18 L20 L21 L22 | A4 L14 | A4 A6 S1 S2 L39 S15 S16 | A5 A6 L13 L20 L21 L22 L24 | A5 A6 S7 S8 L38 S9 | A6 L18 L19 L20 | A6 L20 L21 L22 | A5 L22 L23 L24 | A5 S8 L38 | A5 A6 S0 S1 S16 S17 S18 | A6 L20 L22 | A5 S0 S18 S19 S20 L40 S21 S22 S23 bodies 1
extrude "Extrude1'''''''" add 6 faces at (11.2946, -1.65, 4.0787) (1.8113, -1.65, 4.6017) (-6.1117, -1.65, 5.2575) (4.1787, -1.65, -3.5547) (6.4496, -1.65, -5.504) (8.7204, -1.65, -7.4533) along direction (0, -1, 0) blind 0.1 separate body on bodies 1 makes body 78 at (6.4496, -1.65, -5.504) makes body 79 at (-6.1117, -1.65, 5.2575) makes body 80 at (11.2946, -1.65, 4.0787) makes body 81 at (1.8113, -1.65, 4.6017) makes body 82 at (4.1787, -1.65, -3.5547) makes body 83 at (8.7204, -1.65, -7.4533) in component "NFC Text"
sketch "Sketch4" plane through (0, 0, 0) normal (0, 1, 0) x (-1, 0, 0)
  circle A0 centre (0, 0) radius 33
  circle A1 centre (0, 0) radius 25
  dimension "d65" = 50
  constraint concentric A0 A1
  measures "d65" diameter of A1
extrude "Extrude12" cut sketch "Sketch4" against normal blind 1.1 from surface at -0.4 contours A1 bodies 1
sketch "Sketch5" plane through (0, 0, 0) normal (0, 1, 0) x (1, 0, 0)
  line L0 (0, 0) -> (-140, 0)
  circle A0 centre (-140, 0) radius 2.75
  circle A1 centre (-140, 0) radius 3.25
  circle A2 centre (-140, 0) radius 8.75
  circle A3 centre (-140, 0) radius 9.25
  circle A4 centre (-140, 0) radius 14.5
  circle A5 centre (-140, 0) radius 15
  circle A6 centre (-140, 0) radius 20
  line L1 (-145.7425, -19.1579) -> (-144.2759, -14.3776)
  line L2 (-142.1402, -8.999) -> (-144.4062, -19.5086)
  line L3 (-141.6763, -9.0969) -> (-143.9426, -19.6076)
  line L4 (-140.0901, -9.2496) -> (-140, -20)
  line L5 (-142.1766, -14.8412) -> (-142.875, -19.7923)
  line L6 (-142.5258, -19.8399) -> (-141.8842, -14.8812)
  line L7 (-141.5359, -14.9212) -> (-142.004, -19.8993)
  line L8 (-141.6278, -19.9336) -> (-141.2196, -14.9503)
  line L9 (-140.892, -14.9735) -> (-141.0851, -19.9705)
  line L10 (-140.7279, -19.9868) -> (-140.5348, -14.9905)
  line L11 (-144.2759, -14.3776) -> (-142.5893, -8.8802)
  line L12 (-139.8052, -3.2442) -> (-138.3, -14.4)
  line L13 (-139.62, -14.495) -> (-139.62, -9.2422)
  line L14 (-133.5996, -13.011) -> (-138.7604, -3.0043)
  line L15 (-138.3137, -2.7783) -> (-133.1543, -12.7823)
  line L16 (-134.9286, -13.5842) -> (-136.7372, -8.6554)
  line L17 (-135.391, -13.748) -> (-137.2006, -8.8162)
  line L18 (-136.7372, -14.1281) -> (-137.856, -8.9981)
  line L19 (-138.6318, -8.6424) -> (-139.3678, -3.1879)
  line L20 (-132.1595, -12.1974) -> (-135.0994, -7.8452)
  line L21 (-131.7337, -11.9129) -> (-134.6727, -7.5619)
  line L22 (-134.4577, -7.4058) -> (-131.1145, -11.4585)
  line L23 (-133.9819, -7.0246) -> (-130.6407, -11.0749)
  line L24 (-133.5892, -6.6681) -> (-129.8253, -10.3308)
  line L25 (-128.4, -8.7) -> (-132.5309, -5.4566)
  line L26 (-126.3934, -5.0109) -> (-131.3557, -3.2923)
  line L27 (-131.1734, -2.7664) -> (-121.041, -6.3684)
  line L28 (-130.8111, -1.061) -> (-120.1041, -2.0381)
  dimension "d69" = 140
  dimension "d70" = 5.5
  dimension "d72" = 17.5
  dimension "d74" = 29
  dimension "d75" = 0.5
  dimension "d76" = 0.5
  dimension "d77" = 0.5
  dimension "d78" = 40
  constraint coincident L0.start origin
  constraint horizontal L0
  constraint coincident L0.end A0.centre
  constraint concentric A1 A2
  constraint concentric A0 A3
  constraint concentric A2 A4
  constraint concentric A1 A5
  constraint concentric A2 A6
  constraint coincident A6 L1.start
  constraint coincident A5 L1.end
  constraint coincident A3 L2.start
  constraint coincident A6 L2.end
  constraint coincident A3 L3.start
  constraint coincident A6 L3.end
  constraint parallel L2 L3
  constraint coincident A3 L4.start
  constraint coincident A6 L4.end
  constraint coincident A5 L5.start
  constraint coincident A6 L5.end
  constraint coincident A6 L6.start
  constraint coincident A5 L6.end
  constraint coincident A5 L7.start
  constraint coincident A6 L7.end
  constraint coincident A6 L8.start
  constraint coincident A5 L8.end
  constraint coincident A5 L9.start
  constraint coincident A6 L9.end
  constraint coincident A6 L10.start
  constraint coincident A5 L10.end
  constraint parallel L9 L10
  constraint coincident A3 L11.end
  constraint parallel L1 L11
  constraint coincident A1 L12.start
  constraint coincident A4 L12.end
  constraint coincident A4 L13.start
  constraint coincident A3 L13.end
  constraint vertical L13
  constraint coincident A4 L14.start
  constraint coincident A1 L14.end
  constraint coincident A1 L15.start
  constraint coincident A4 L15.end
  constraint parallel L14 L15
  constraint coincident A4 L16.start
  constraint coincident A3 L16.end
  constraint coincident A4 L17.start
  constraint coincident A3 L17.end
  constraint parallel L16 L17
  constraint coincident A4 L18.start
  constraint coincident A3 L18.end
  constraint coincident A2 L19.start
  constraint coincident A1 L19.end
  constraint parallel L12 L19
  constraint coincident A4 L20.start
  constraint coincident A3 L20.end
  constraint coincident A4 L21.start
  constraint coincident A3 L21.end
  constraint parallel L20 L21
  constraint coincident A3 L22.start
  constraint coincident A4 L22.end
  constraint coincident A3 L23.start
  constraint coincident A4 L23.end
  constraint parallel L22 L23
  constraint coincident A3 L24.start
  constraint coincident A4 L24.end
  constraint coincident A4 L25.start
  constraint coincident A3 L25.end
  constraint coincident A4 L26.start
  constraint coincident A3 L26.end
  constraint coincident A3 L27.start
  constraint coincident A6 L27.end
  constraint coincident A3 L28.start
  constraint coincident A6 L28.end
  measures "d69" distance of L0.start L0.end
  measures "d70" diameter of A0
  measures "d72" diameter of A2
  measures "d74" diameter of A4
  measures "d75" distance of A4 A5
  measures "d76" distance of A0 A1
  measures "d77" distance of A2 A3
  measures "d78" diameter of A6
component "Ring 0 - pro" placed x (1, 0, 0) y (0, 1, 0) z (0, 0, 1) at (0, 0, 0)
component "Ring 0 - con" placed x (1, 0, 0) y (0, 1, 0) z (0, 0, 1) at (0, 0, 0)
component "Ring 1 - pro" placed x (1, 0, 0) y (0, 1, 0) z (0, 0, 1) at (0, 0, 0)
component "Ring 1 - con" placed x (1, 0, 0) y (0, 1, 0) z (0, 0, 1) at (0, 0, 0)
component "Ring 2 - pro" placed x (1, 0, 0) y (0, 1, 0) z (0, 0, 1) at (0, 0, 0)
component "Ring 2 - con" placed x (1, 0, 0) y (0, 1, 0) z (0, 0, 1) at (0, 0, 0)
component "Thesis" placed x (1, 0, 0) y (0, 1, 0) z (0, 0, 1) at (0, 0, 0)
component "NFC Text" placed x (1, 0, 0) y (0, 1, 0) z (0, 0, 1) at (0, 0, 0)
equation "d21 = 24 mm"
equation "d22 = d21 - 3 mm"
equation "d23 = d22 - 3 mm"
equation "d24 = d23 - 3 mm"
equation "d25 = d24 - 3 mm"
equation "d26 = d25 - 3 mm"
equation "d32 = ( 35 * 1.6 ) * 1 mm"
equation "d75 = d77"
equation "d77 = d76"
